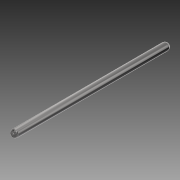
# Autodesk Inventor part: EjeMotor
Saved by Autodesk Inventor 2013 (Build 170138000, 138)
## iProperties
Created: 2013-06-25
Part Number: EjeMotor
Material: Genérico
Document SubType Name: Modeling
Designer: usuario
Density: 1 g/cm^3
Author: usuario
Autodesk Inventor part; units mm, degrees
ref_plane "YZ Plane" through (0, 0, 0) normal (1, 0, 0) x (0, 1, 0)
ref_plane "XZ Plane" through (0, 0, 0) normal (0, 1, 0) x (-1, 0, 0)
ref_plane "XY Plane" through (0, 0, 0) normal (0, 0, 1) x (1, 0, 0)
sketch "Boceto1" plane through (0, 0, 0) normal (0, 1, 0) x (-1, 0, 0)
  circle A0 centre (0, 0) radius 1
  dimension "d0" = 2
  constraints: 1 centre point, 1 coincident
  measures "d0" diameter of A0
extrude "Extrusión1" add sketch "Boceto1" along normal mid plane 40.91
sketch "Boceto2" plane through (0, 20.455, 0) normal (0, 1, 0) x (1, 0, 0)
  circle A0 centre (0, 0) radius 1 projected
  circle A1 centre (0, 0) radius 1
  line L0 (1, 0) -> (-1, 0)
  constraints: 2 end point, 2 point on circle, 1 centre point, 1 coincident, 1 horizontal alignment, 1 midpoint, 2 other
revolve "Revolución1" add sketch "Boceto2" angle 360 about axis through (1, 20.455, 0) along (-1, 0, 0) picked at (0.2495, 0.221) contours L0 A0
sketch "Boceto3" plane through (0, -20.455, 0) normal (0, -1, 0) x (1, 0, 0)
  circle A0 centre (0, 0) radius 1 projected
  circle A1 centre (0, 0) radius 1
  line L0 (1, 0) -> (-1, 0)
  constraints: 2 end point, 2 point on circle, 1 centre point, 1 coincident, 1 horizontal alignment, 1 midpoint, 2 other
revolve "Revolución2" add sketch "Boceto3" angle 360 about axis through (1, -20.455, 0) along (-1, 0, 0) picked at (0.2495, 0.221) contours L0 A0
